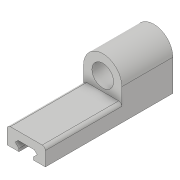
# Autodesk Inventor part: Laser mount 5 inches
Saved by Autodesk Inventor 2019 (Build 230136000, 136)
## iProperties
Created: 2019-10-18
Part Number: Laser mount 5 inches
Material: Generic
Document SubType Name: Modeling
Designer: wrexroat
Density: 1 g/cm^3
Appearance: Default
Author: wrexroat
Autodesk Inventor part; units mm, degrees
ref_plane "YZ Plane" through (0, 0, 0) normal (1, 0, 0) x (0, 1, 0)
ref_plane "XZ Plane" through (0, 0, 0) normal (0, 1, 0) x (-1, 0, 0)
ref_plane "XY Plane" through (0, 0, 0) normal (0, 0, 1) x (1, 0, 0)
sketch "Sketch1" plane through (0, 0, 0) normal (0, 0, 1) x (1, 0, 0)
  line L0 (-7.2739, -1.4271) -> (7.2739, -1.4271)
  line L1 (7.2739, -1.4271) -> (7.2739, 1.4271)
  line L2 (7.2739, 1.4271) -> (-7.2739, 1.4271)
  line L3 (-7.2739, 1.4271) -> (-7.2739, -1.4271)
  line L4 (-7.2739, -1.4271) -> (7.2739, 1.4271) construction
  line L5 (7.2739, -1.4271) -> (-7.2739, 1.4271) construction
  line L6 (9.525, 3.6783) -> (-9.525, 3.6783)
  line L7 (-9.525, 3.6783) -> (-9.525, 6.4723)
  line L8 (-9.525, 6.4723) -> (9.525, 6.4723)
  line L9 (9.525, 6.4723) -> (9.525, 3.6783)
  line L10 (9.525, 3.6783) -> (-9.525, 6.4723) construction
  line L11 (-9.525, 3.6783) -> (9.525, 6.4723) construction
  line L12 (-7.2739, 1.4271) -> (-9.525, 3.6783)
  line L13 (7.2739, 1.4271) -> (9.525, 3.6783)
  line L14 (-10.922, 5.0753) -> (-8.1026, 7.8947)
  line L15 (-10.922, 5.0753) -> (-6.9348, 5.0753) construction
  line L16 (-10.922, 5.0753) -> (-9.525, 3.6783)
  line L17 (10.922, 5.0753) -> (8.1026, 7.8947)
  line L18 (9.525, 3.6783) -> (10.922, 5.0753)
  line L19 (-8.1026, 7.8947) -> (8.1026, 7.8947)
  line L20 (-19.05, -1.4271) -> (19.05, -1.4271)
  line L21 (19.05, -1.4271) -> (19.05, 15.8839)
  line L22 (19.05, 15.8839) -> (-19.05, 15.8839)
  line L23 (-19.05, 15.8839) -> (-19.05, -1.4271)
  point P0 (0, 0)
  point P1 (0, 5.0753)
  point P2 (0, -1.4271)
  dimension "d0" = 135
  dimension "d1" = 135
  dimension "d2" = 19.05
  dimension "d3" = 2.794
  dimension "d4" = 45
  dimension "d5" = 4.2164
  dimension "d6" = 90
  dimension "d7" = 90
  dimension "d8" = 9.3218
  dimension "d9" = 38.1
  constraints: 48 end point, 7 parallel, 6 midpoint, 5 horizontal, 4 perpendicular, 2 point on line, 1 equal length
  measures "d0" angle of L3 L12
  measures "d1" angle of L1 L13
  measures "d2" distance between parallel lines of L9 L7
  measures "d3" distance of L6.end L7.end
  measures "d4" angle of L15 L14
  measures "d5" distance between parallel lines of L19 L6
  measures "d6" angle of L18 L17
  measures "d7" angle of L16 L14
  measures "d8" distance between parallel lines of L0 L19
  measures "d9" distance of L21.end L22.end
extrude "Extrusion1" add sketch "Sketch1" against normal blind 177.8 contours L20 L23 L22 L21 L1 L13 L18 L17 L19 L14 L16 L12 L3
sketch "Sketch2" plane through (0, 0, -177.8) normal (0, 0, -1) x (-1, 0, 0)
  arc A0 (19.05, 29.7163) -> (-19.05, 29.7163) centre (0, 29.7163) ccw
  line L0 (19.05, -1.4271) -> (19.05, 15.8839) projected
  line L1 (19.05, 15.8839) -> (19.05, -1.4271) projected
  line L2 (19.05, 15.8839) -> (19.05, 29.7163)
  line L3 (-19.05, -1.4271) -> (-19.05, 15.8839) projected
  line L4 (-19.05, 15.8839) -> (-19.05, 29.7163)
  line L5 (19.05, 15.8839) -> (-19.05, 15.8839)
  point P0 (0, 0)
  constraints: 6 end point, 3 tangent, 2 point on circle, 1 centre point, 1 perpendicular
extrude "Extrusion2" add sketch "Sketch2" against normal blind 50.8
sketch "Sketch3" plane through (0, 0, -177.8) normal (0, 0, -1) x (-1, 0, 0)
  arc A0 (19.05, 29.7163) -> (-19.05, 29.7163) centre (0, 29.7163) ccw projected
  point P0 (0, 0)
  constraints: 1 coincident
hole "Hole1" at (0, 29.7163, -177.8) direction (0, 0, 1) diameter 21.6 end through all
fillet "Fillet1" radius 3.175 2 edges at (-19.05, 15.8839, -63.5) (19.05, 15.8839, -63.5)
sketch "Sketch4" plane through (0, 0, 0) normal (0, 0, 1) x (1, 0, 0)
  line L0 (-84.0587, 46.9015) -> (30.6415, 46.9015)
  line L1 (30.6415, 46.9015) -> (30.6415, -6.8679)
  line L2 (30.6415, -6.8679) -> (-84.0587, -6.8679)
  line L3 (-84.0587, -6.8679) -> (-84.0587, 46.9015)
  line L4 (-84.0587, 46.9015) -> (30.6415, -6.8679) construction
  line L5 (30.6415, 46.9015) -> (-84.0587, -6.8679) construction
  point P0 (0, 0)
  point P1 (-26.7086, 20.0168)
  constraints: 12 end point, 2 midpoint, 2 parallel, 1 horizontal, 1 perpendicular
extrude "Extrusion3" cut sketch "Sketch4" against normal blind 50.8
body "Solid1"
